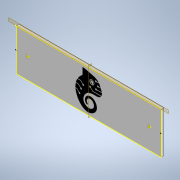
# Autodesk Inventor part: wooden_backcover
Saved by Autodesk Inventor 2020 (Build 240168000, 168)
## iProperties
Created: 2019-07-26
Part Number: wooden_backcover
Material: Generic
Document SubType Name: Modeling
Designer: erwin
Density: 1 g/cm^3
Appearance: Default
Mass: 1273.68 g
Surface Area: 2310.96 cm^2
Volume: 1273.68 cm^3
Author: erwin
Autodesk Inventor part; units mm, degrees
ref_plane "YZ Plane" through (0, 0, 0) normal (1, 0, 0) x (0, 1, 0)
ref_plane "XZ Plane" through (0, 0, 0) normal (0, 1, 0) x (-1, 0, 0)
ref_plane "XY Plane" through (0, 0, 0) normal (0, 0, 1) x (1, 0, 0)
ref_plane "Work Plane1" through (0, 0, 0) normal (0, 0, 1) x (1, 0, 0)
sketch "Sketch1" plane through (0, 0, 0) normal (0, 0, 1) x (1, 0, 0)
  line L0 (612, -44.7721) -> (612, -100.7605) projected
  line L1 (0, 0) -> (612, 0) projected
  line L2 (612, -176) -> (0, -176) projected
  line L3 (612, 0) -> (0, 0)
  line L4 (0, 0) -> (0, -176)
  line L5 (0, -176) -> (612, -176)
  line L6 (612, -176) -> (612, 0)
  constraints: 8 end point, 2 parallel, 1 horizontal, 1 perpendicular
extrude "Extrusion1" add sketch "Sketch1" against normal blind 12
thicken "Thicken1" operation add thickness 1 both sides no extend neighbours yes toward (1, 0, 0) faces at (0, -58.6667, -4) (204, -176, -4) (612, -29.8481, -4) (612, -82.0977, -4) (612, -150.9202, -4) (408, 0, -4)
sketch "Sketch2" plane through (0, 0, 0) normal (0, 0, 1) x (1, 0, 0)
  circle A0 centre (51, -88) radius 4
  line L0 (611, -1) -> (1, -1) projected
  line L1 (1, -175) -> (611, -175) projected
  line L2 (1, -1) -> (1, -175) projected
  point P0 (0, 0)
  dimension "d4" = 8
  dimension "d5" = 87
  dimension "d6" = 87
  dimension "d7" = 50
  constraints: 1 centre point
  measures "d4" diameter of A0
  measures "d5" distance from line of L0 A0.centre
  measures "d6" distance from line of L1 A0.centre
  measures "d7" distance from line of L2 A0.centre
extrude "Extrusion2" cut sketch "Sketch2" against normal blind 12
ref_plane "Work Plane2" through (306, -175, 0) normal (-1, 0, 0) x (0, 0, 1)
mirror "Mirror1" about plane through (306, -175, 0) normal (-1, 0, 0) of "Extrusion2"
sketch "Sketch3" plane through (0, 0, 0) normal (0, 0, 1) x (1, 0, 0)
  line L0 (1, -1) -> (611, -1) construction
  line L1 (611, -1) -> (611, -175) construction
  line L2 (611, -175) -> (1, -175) construction
  line L3 (1, -175) -> (1, -1) construction
  line L4 (611, -175) -> (611, -1) projected
  line L5 (1, -1) -> (1, -175) projected
  point P0 (0, 0)
  point P1 (611, -88)
  point P2 (1, -88)
  constraints: 4 midpoint, 1 point on line, 2 other
sketch "Sketch4" plane through (0, 0, 0) normal (0, 0, 1) x (1, 0, 0)
  circle A0 centre (561, -88) radius 4 projected
  circle A1 centre (51, -88) radius 4 projected
  line L0 (611, -175) -> (611, -1) projected
  line L1 (611, -1) -> (1, -1) projected
  line L2 (1, -1) -> (1, -175) projected
  line L3 (1, -175) -> (611, -175) projected
  point P0 (0, 0)
equation "\"d5\" = d6"
body "Solid1"
